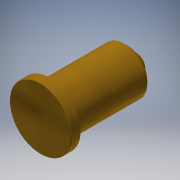
# Autodesk Inventor part: Pogo-pin
Saved by Autodesk Inventor 2017 (Build 210142000, 142)
## iProperties
Created: 2018-07-06
Part Number: Pogo-pin
Material: Generic
Document SubType Name: Modeling
Designer: intelsath
Density: 1 g/cm^3
Appearance: Default
Author: intelsath
Autodesk Inventor part; units mm, degrees
ref_plane "YZ Plane" through (0, 0, 0) normal (1, 0, 0) x (0, 1, 0)
ref_plane "XZ Plane" through (0, 0, 0) normal (0, 1, 0) x (-1, 0, 0)
ref_plane "XY Plane" through (0, 0, 0) normal (0, 0, 1) x (1, 0, 0)
sketch "Sketch1" plane through (0, 0, 0) normal (0, 0, 1) x (1, 0, 0)
  line L0 (0, 0) -> (0.98, 0)
  line L1 (0.98, 0) -> (1, 0.02)
  line L2 (1, 0.02) -> (1, 0.3)
  line L3 (1, 0.3) -> (0.75, 0.3)
  line L4 (0.75, 0.3) -> (0.75, 2.7)
  line L5 (0.75, 2.7) -> (0.65, 2.8)
  line L6 (0.65, 2.8) -> (0.45, 2.8)
  line L7 (0.45, 2.8) -> (0.45, 2.755)
  arc A0 (0.45, 2.755) -> (0, 3.205) centre (0, 2.755) ccw
  line L8 (0, 3.205) -> (0, 0)
  dimension "d0" = 135
  dimension "d1" = 45
  dimension "d2" = 0.45
  dimension "d3" = 1
  dimension "d4" = 0.02
  dimension "d5" = 0.1
  dimension "d6" = 0.75
  dimension "d7" = 3.205
  dimension "d8" = 2.8
  dimension "d9" = 0.3
  constraints: 18 end point, 4 perpendicular, 2 point on circle, 1 centre point, 1 horizontal, 1 parallel, 1 point on line, 1 tangent, 1 vertical
  measures "d0" angle of L0 L1
  measures "d1" angle of L4 L5
  measures "d2" radius of A0
  measures "d3" distance between parallel lines of L8 L2
  measures "d4" distance from line of L0.end L2
  measures "d5" horizontal distance of L4.end L5.end
  measures "d6" distance between parallel lines of L8 L4
  measures "d7" distance of L8.start L0.start
  measures "d8" distance between parallel lines of L0 L6
  measures "d9" distance between parallel lines of L0 L3
revolve "Revolution1" add sketch "Sketch1" angle 360 about axis through (0, 3.205, 0) along (0, -1, 0)
body "Solid1"
